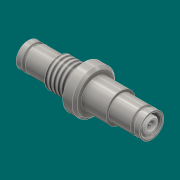
# Autodesk Inventor part: shv
Saved by Autodesk Inventor 2016 SP1 (Build 200210100, 210)
## iProperties
Created: 2016-04-02
Part Number: shv
Material: Steel, Alloy
Document SubType Name: Modeling
Designer: sawai
Density: 7.73 g/cm^3
Appearance: Semi-Polished
Author: sawai
Title: KINGS  1709-1
Comments: http://www.newark.com/kings/1709-1/rf-coaxial-adapter-shv-plug-shv/dp/93F6329
Autodesk Inventor part; units mm, degrees
ref_plane "YZ Plane" through (0, 0, 0) normal (1, 0, 0) x (0, 1, 0)
ref_plane "XZ Plane" through (0, 0, 0) normal (0, 1, 0) x (-1, 0, 0)
ref_plane "XY Plane" through (0, 0, 0) normal (0, 0, 1) x (1, 0, 0)
sketch "Sketch1" plane through (0, 0, 0) normal (1, 0, 0) x (0, 1, 0)
  circle A0 centre (0, 0) radius 8.763
  dimension "d0" = 17.526
  constraints: 1 centre point, 1 coincident
  measures "d0" diameter of A0
extrude "Extrusion1" add sketch "Sketch1" along normal mid plane 50.546
sketch "Sketch2" plane through (25.273, 0, 0) normal (1, 0, 0) x (0, 0, -1)
  circle A0 centre (0, 0) radius 5
  circle A1 centre (0, 0) radius 8.763 projected
  dimension "d3" = 10
  constraints: 1 centre point, 1 coincident
  measures "d3" diameter of A0
extrude "Extrusion2" cut sketch "Sketch2" against normal blind 12.7
sketch "Sketch3" plane through (12.573, 0, 0) normal (1, 0, 0) x (0, 0, -1)
  circle A0 centre (0, 0) radius 5 projected
  circle A1 centre (0, 0) radius 8.763 projected
  circle A2 centre (0, 0) radius 6
  dimension "d6" = 1
  constraints: 1 centre point
  measures "d6" radial gap between concentric circles of A0 A2
extrude "Extrusion3" cut sketch "Sketch3" against normal blind 10.16 contours A1
sketch "Sketch4" plane through (25.273, 0, 0) normal (1, 0, 0) x (0, 0, -1)
  circle A0 centre (0, 0) radius 5 projected
  circle A1 centre (0, 0) radius 0.5
  circle A2 centre (0, 0) radius 4
  dimension "d9" = 1
  dimension "d10" = 1
  constraints: 2 centre point, 1 coincident
  measures "d9" diameter of A1
  measures "d10" radial gap between concentric circles of A0 A2
extrude "Extrusion4" cut sketch "Sketch4" against normal blind 17.78 contours A2
chamfer "Chamfer1" distance 0.4 angle 45 2 edges at (25.273, 0, 0.5) (25.273, 0, 4)
mirror "Mirror2" about plane through (0, 0, 0) normal (1, 0, 0) of "Extrusion2", "Extrusion3", "Extrusion4"
chamfer "Chamfer2" distance 0.4 angle 45 2 edges at (-25.273, 0, 4) (-25.273, 0, 0.5)
thread "Thread1" size "M12x1.75" class "6g" standard "ANSI Metric M Profile" full length
sketch "Sketch5" plane through (0, 0, 0) normal (0, 1, 0) x (-1, 0, 0)
  line L0 (-12.573, 5) -> (-12.573, -5) projected
  line L1 (-25.273, 5) -> (-25.273, -5) projected
  line L2 (-25.273, 5) -> (-12.573, 5) projected
  circle A0 centre (-22.273, 5) radius 0.75
  line L3 (35.3822, 0) -> (-35.3822, 0) projected
  point P0 (0, 0)
  dimension "d21" = 1.5
  dimension "d22" = 3
  constraints: 1 centre point, 1 point on line
  measures "d21" diameter of A0
  measures "d22" distance from line of L1 A0.centre
revolve "Revolution1" cut sketch "Sketch5" angle 360 about axis through (-10, 0, 0) along (1, 0, 0) contours A0 L2 | L2 A0
mirror "Mirror3" about plane through (0, 0, 0) normal (1, 0, 0) of "Revolution1"
chamfer "Chamfer3" distance 1 angle 45 1 edges at (2.413, -8.763, 0)
sketch "Sketch6" plane through (7.493, 0, 0) normal (1, 0, 0) x (0, 0, -1)
  circle A0 centre (0, 0) radius 4 projected
  circle A1 centre (0, 0) radius 3
  circle A2 centre (0, 0) radius 1.5
  dimension "d27" = 1
  dimension "d28" = 1.5
  constraints: 2 centre point
  measures "d27" radial gap between concentric circles of A0 A1
  measures "d28" radial gap between concentric circles of A1 A2
extrude "Extrusion5" add sketch "Sketch6" along normal up to surface (17.78 mm away) separate body contours A1
mirror "Mirror4" about plane through (0, 0, 0) normal (1, 0, 0) of "Extrusion5" bodies 2
chamfer "Chamfer4" distance 0.5 angle 45 2 edges at (25.273, 0, 1.5) (25.273, 0, 3)
chamfer "Chamfer5" distance 0.5 angle 45 2 edges at (-25.273, 0, 1.5) (-25.273, 0, 3)
body "Solid1"
body "Solid2"
